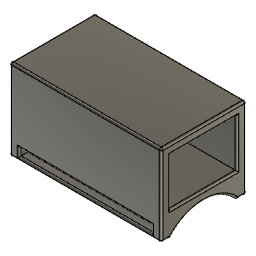
CPS_Lab_Enclosure v3_new (Autodesk Fusion 360 design; units mm, degrees)
Autodesk Fusion 360 part; units mm, degrees
sketch "Sketch2" plane through (0, 0, 0) normal (0, 0, 1) x (1, 0, 0)
  line L0 (0, 0) -> (80, 0)
  line L1 (80, 0) -> (80, -45)
  line L2 (80, -45) -> (0, -45)
  line L3 (0, -45) -> (0, 0)
  line L4 (0, 0) -> (5, 0)
  line L5 (5, -5) -> (5, -40)
  line L6 (5, -5) -> (75, -5)
  line L7 (5, -5) -> (80, -5)
  line L8 (80, -40) -> (5, -40)
  line L9 (5, -40) -> (5, -5)
  dimension "d1" = 80
  dimension "d2" = 45
  dimension "d3" = 70
  dimension "d4" = 35
  constraint horizontal L0
  constraint vertical L1
  constraint horizontal L2
  constraint vertical L3
  constraint coincident L0.start L3.end
  constraint coincident L0 L4.end
  constraint perpendicular L2 L5
  constraint perpendicular L1 L6
  constraint horizontal L7
  constraint horizontal L8
  constraint vertical L9
  constraint coincident L1 L7.end
  constraint coincident L6.end L7
  constraint coincident L1 L8.start
  measures "d1" distance of L0.start L0.end
  measures "d2" distance of L0.start L2.end
  measures "d3" distance of L5.start L6.end
  measures "d4" distance of L5.start L5.end
extrude "Extrude1" add sketch "Sketch2" along normal blind 35
extrude "Extrude2" cut sketch "Sketch2" along normal blind 25 from surface at 5 contours L1 L5 L6 L7 L8 L9
sketch "Sketch3" plane through (0, -45, 0) normal (0, -1, 0) x (1, 0, 0)
  line L0 (0, 0) -> (80, 0)
  line L1 (80, 0) -> (80, 35)
  line L2 (80, 35) -> (0, 35)
  line L3 (0, 35) -> (0, 0)
  line L4 (0, 0) -> (80, 0)
  line L5 (80, 0) -> (80, -8)
  line L6 (80, -8) -> (0, -8)
  line L7 (0, -8) -> (0, 0)
  line L8 (5, -6) -> (75, -6)
  line L9 (75, -6) -> (75, -2)
  line L10 (75, -2) -> (5, -2)
  line L11 (5, -2) -> (5, -6)
  dimension "d10" = 8
  dimension "d11" = 70
  constraint horizontal L4
  constraint vertical L5
  constraint horizontal L6
  constraint vertical L7
  constraint coincident L0.start L3.end
  constraint horizontal L8
  constraint vertical L9
  constraint horizontal L10
  constraint vertical L11
  measures "d10" distance of L0.start L6.end
  measures "d11" distance of L8.start L8.end
extrude "Extrude3" add sketch "Sketch3" against normal blind 5 contours L0 L4 L5 L6 L7
sketch "Sketch4" plane through (0, 0, 0) normal (0, 1, 0) x (-1, 0, 0)
  line L0 (-80, 0) -> (0, 0)
  line L1 (0, 0) -> (0, 35)
  line L2 (0, 35) -> (-80, 35)
  line L3 (-80, 35) -> (-80, 0)
  line L4 (-80, 0) -> (0, 0)
  line L5 (0, 0) -> (0, -8)
  line L6 (0, -8) -> (-80, -8)
  line L7 (-80, -8) -> (-80, 0)
  line L8 (-75, -2) -> (-5, -2)
  line L9 (-5, -2) -> (-5, -6)
  line L10 (-5, -6) -> (-75, -6)
  line L11 (-75, -6) -> (-75, -2)
  constraint horizontal L4
  constraint vertical L5
  constraint horizontal L6
  constraint vertical L7
  constraint coincident L0.start L3.end
  constraint horizontal L8
  constraint vertical L9
  constraint horizontal L10
  constraint vertical L11
extrude "Extrude4" add sketch "Sketch4" against normal blind 5 contours L0 L4 L5 L6 L7
sketch "Sketch5" plane through (5, 0, 0) normal (1, 0, 0) x (0, 1, 0)
  line L0 (-40, 5) -> (-5, 5)
  line L1 (-5, 5) -> (-5, 30)
  line L2 (-5, 30) -> (-40, 30)
  line L3 (-40, 30) -> (-40, 5)
  line L4 (-40, -8) -> (-5, -8)
  line L5 (-22.5, -8) -> (-22.5, 0)
  arc A0 (-5, -8) -> (-40, -8) centre (-22.5, -23.1406) ccw
  line L6 (-40, 0) -> (-5, 0)
  line L7 (-5, 0) -> (-5, -8)
  line L8 (-5, -8) -> (-40, -8)
  line L9 (-40, -8) -> (-40, 0)
  constraint horizontal L4
  constraint midpoint L4 L5.start
  constraint perpendicular L4 L5
  constraint coincident L5.end A0
  constraint horizontal L6
  constraint vertical L7
  constraint horizontal L8
  constraint vertical L9
extrude "Extrude5" add sketch "Sketch5" along normal blind 80 from surface at -5 contours A0 L6 L9 | A0 L6 L7
extrude "Extrude6" cut sketch "Sketch4" along normal through all and the other way through all contours L8 L9 L10 L11
fillet "Fillet1" radius 1 8 faces at (80, -4.1117, -2.8872) (26.6667, -26.8832, -0.4189) (26.6667, -1.6667, -8) (53.3333, -43.3333, -8) (28.3333, 0, 22.6667) (26.6667, -15, 35) (28.3333, -45, 22.6667) (0, -22.5, 23.3333)
